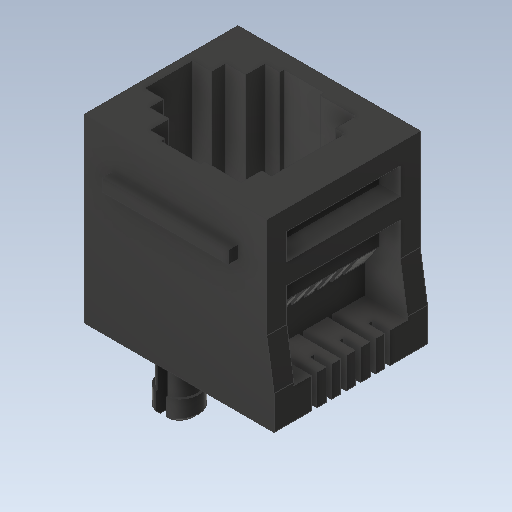
# Autodesk Inventor part: RJ12 - Straight
Saved by Autodesk Inventor 2020 (Build 240168000, 168)
## iProperties
Created: 2017-10-30
Part Number: RJ12 - Straight
Material: Thermoplastic Resin
Document SubType Name: Modeling
Designer: Alex
Density: 1.28 g/cm^3
Appearance: Smooth - Black
Mass: 2.13301 g
Surface Area: 25.086 cm^2
Volume: 1.66642 cm^3
Catalog Web Link: https://www.digikey.com/product-detail/en/assmann-wsw-components/A-2014-1-4-N-T-R/AE10395-ND/2183646
Description: Board Mount RJ12 - Straight
Vendor: Digikey
Author: Alex
Autodesk Inventor part; units mm, degrees
ref_plane "YZ Plane" through (0, 0, 0) normal (1, 0, 0) x (0, 1, 0)
sketch "Sketch1" plane through (0, 0, 0) normal (0, 1, 0) x (-1, 0, 0)
  line L0 (7.9375, -6.6802) -> (-7.9375, -6.6802)
  line L1 (-7.9375, -6.6802) -> (-7.9375, 6.6802)
  line L2 (-7.9375, 6.6802) -> (7.9375, 6.6802)
  line L3 (7.9375, 6.6802) -> (7.9375, -6.6802)
  line L4 (7.9375, -6.6802) -> (-7.9375, 6.6802) construction
  line L5 (-7.9375, -6.6802) -> (7.9375, 6.6802) construction
  point P0 (0, 0)
  dimension "d0" = 15.875
  dimension "d1" = 13.3604
  constraints: 12 end point, 2 midpoint, 2 parallel, 1 horizontal, 1 perpendicular
  measures "d0" distance of L1.end L2.end
  measures "d1" distance of L0.end L1.end
extrude "Extrusion1" add sketch "Sketch1" along normal blind 15.748
sketch "Sketch2" plane through (-7.9375, 0, 6.6802) normal (0, 0, 1) x (1, 0, 0)
  line L0 (15.875, 0) -> (15.875, 15.748) projected
  line L1 (15.875, 0) -> (16.51, 0)
  line L2 (16.51, 0) -> (16.51, 2.921)
  line L3 (16.51, 2.921) -> (15.875, 6.9596)
  line L4 (15.875, 0) -> (15.875, 6.9596)
  line L5 (0, 0) -> (0, 15.748) projected
  line L6 (0, 15.748) -> (15.875, 15.748) projected
  point P0 (7.9375, 0)
  dimension "d4" = 16.51
  dimension "d5" = 2.921
  dimension "d6" = 8.7884
  constraints: 8 end point, 1 horizontal, 1 parallel, 1 perpendicular, 1 point on line
  measures "d4" distance between parallel lines of L5 L2
  measures "d5" distance of L1.end L2.end
  measures "d6" distance from line of L6 L3.end
extrude "Extrusion2" add sketch "Sketch2" against normal up to surface (13.3604 mm away)
sketch "Sketch3" plane through (0, 15.748, 0) normal (0, 1, 0) x (1, 0, 0)
  line L0 (-7.3025, -2.1082) -> (-5.6515, -2.1082)
  line L1 (-5.6515, -2.1082) -> (-5.6515, -3.3401)
  line L2 (-5.6515, -3.3401) -> (-3.9243, -3.3401)
  line L3 (-3.9243, -3.3401) -> (-3.9243, -5.0292)
  line L4 (-3.9243, -5.0292) -> (-2.6289, -5.0292)
  line L5 (-2.6289, -5.0292) -> (-2.6289, -5.3975)
  line L6 (-2.6289, -5.3975) -> (0.8763, -5.3975)
  line L7 (0.8763, -5.3975) -> (0.8763, -5.0292)
  line L8 (0.8763, -5.0292) -> (4.0513, -5.0292)
  line L9 (4.0513, -5.0292) -> (4.0513, -3.2131)
  line L10 (4.0513, -3.2131) -> (4.8895, -3.2131)
  line L11 (4.8895, -3.2131) -> (4.8895, 0)
  line L12 (-7.3025, -2.1082) -> (-7.3025, 0)
  line L13 (-7.9375, 6.6802) -> (-7.9375, -6.6802) projected
  line L14 (-7.3025, 0) -> (4.8895, 0) construction
  line L15 (7.9375, -6.6802) -> (7.9375, 6.6802) construction
  line L16 (-7.3025, 2.1082) -> (-5.6515, 2.1082)
  line L17 (-5.6515, 2.1082) -> (-5.6515, 3.3401)
  line L18 (-5.6515, 3.3401) -> (-3.9243, 3.3401)
  line L19 (-3.9243, 3.3401) -> (-3.9243, 5.0292)
  line L20 (-3.9243, 5.0292) -> (-2.6289, 5.0292)
  line L21 (-2.6289, 5.0292) -> (-2.6289, 5.3975)
  line L22 (-2.6289, 5.3975) -> (0.8763, 5.3975)
  line L23 (0.8763, 5.3975) -> (0.8763, 5.0292)
  line L24 (0.8763, 5.0292) -> (4.0513, 5.0292)
  line L25 (4.0513, 5.0292) -> (4.0513, 3.2131)
  line L26 (4.0513, 3.2131) -> (4.8895, 3.2131)
  line L27 (4.8895, 3.2131) -> (4.8895, 0)
  line L28 (-7.3025, 2.1082) -> (-7.3025, 0)
  point P0 (0, 0)
  dimension "d9" = 0.635
  dimension "d10" = 2.1082
  dimension "d11" = 3.048
  dimension "d12" = 0.8382
  dimension "d13" = 3.175
  dimension "d14" = 3.2131
  dimension "d15" = 5.0292
  dimension "d16" = 5.3975
  dimension "d17" = 1.651
  dimension "d18" = 1.7272
  dimension "d19" = 1.2954
  dimension "d20" = 3.5052
  dimension "d21" = 3.3401
  constraints: 54 end point, 12 symmetric about line, 11 perpendicular, 5 point on line, 1 horizontal, 1 parallel
  measures "d9" distance between parallel lines of L13 L12
  measures "d10" distance between parallel lines of L14 L0
  measures "d11" distance between parallel lines of L15 L11
  measures "d12" distance of L9.end L10.end
  measures "d13" distance of L7.end L8.end
  measures "d14" distance between parallel lines of L14 L10
  measures "d15" distance between parallel lines of L14 L8
  measures "d16" distance between parallel lines of L14 L6
  measures "d17" distance of L0.start L0.end
  measures "d18" distance of L1.end L2.end
  measures "d19" distance of L3.end L4.end
  measures "d20" distance of L5.end L6.end
  measures "d21" distance between parallel lines of L14 L2
extrude "Extrusion3" cut sketch "Sketch3" against normal blind 13.97
sketch "Sketch4" plane through (0, 0, 0) normal (1, 0, 0) x (0, 1, 0)
  line L0 (0, 6.6802) -> (15.748, 6.6802) projected
  line L1 (11.5316, 6.6802) -> (12.6492, 6.6802)
  line L2 (12.6492, 6.6802) -> (12.6492, 7.5692)
  line L3 (12.6492, 7.5692) -> (11.5316, 7.5692)
  line L4 (11.5316, 7.5692) -> (11.5316, 6.6802)
  line L5 (15.748, -6.6802) -> (15.748, 6.6802) projected
  line L6 (0, 0) -> (24.5058, 0) construction
  line L7 (11.5316, -6.6802) -> (12.6492, -6.6802)
  line L8 (12.6492, -6.6802) -> (12.6492, -7.5692)
  line L9 (12.6492, -7.5692) -> (11.5316, -7.5692)
  line L10 (11.5316, -7.5692) -> (11.5316, -6.6802)
  dimension "d24" = 1.1176
  dimension "d25" = 3.0988
  dimension "d27" = 7.5692
  constraints: 18 end point, 4 symmetric about line, 2 horizontal, 2 parallel, 1 perpendicular, 1 point on line
  measures "d24" distance of L2.end L3.end
  measures "d25" distance between parallel lines of L5 L2
  measures "d27" distance between parallel lines of L6 L3
extrude "Extrusion4" add sketch "Sketch4" along normal mid plane 10.922
sketch "Sketch5" plane through (0, 0, 0) normal (0, -1, 0) x (1, 0, 0)
  line L0 (-3.2893, 2.8702) -> (3.5687, 2.8702)
  line L1 (3.5687, 2.8702) -> (3.5687, 2.3622)
  line L2 (3.5687, 2.3622) -> (-3.2893, 2.3622)
  line L3 (-3.2893, 2.3622) -> (-3.2893, 2.8702)
  line L4 (8.5725, 6.6802) -> (-7.9375, 6.6802) projected
  line L5 (-7.9375, 6.6802) -> (-7.9375, -6.6802) projected
  line L6 (-3.2893, 1.8542) -> (3.5687, 1.8542)
  line L7 (3.5687, 1.8542) -> (3.5687, 1.3462)
  line L8 (3.5687, 1.3462) -> (-3.2893, 1.3462)
  line L9 (-3.2893, 1.3462) -> (-3.2893, 1.8542)
  line L10 (-3.2893, 0.8382) -> (3.5687, 0.8382)
  line L11 (3.5687, 0.8382) -> (3.5687, 0.3302)
  line L12 (3.5687, 0.3302) -> (-3.2893, 0.3302)
  line L13 (-3.2893, 0.3302) -> (-3.2893, 0.8382)
  line L14 (-3.2893, -0.1778) -> (3.5687, -0.1778)
  line L15 (3.5687, -0.1778) -> (3.5687, -0.6858)
  line L16 (3.5687, -0.6858) -> (-3.2893, -0.6858)
  line L17 (-3.2893, -0.6858) -> (-3.2893, -0.1778)
  line L18 (-3.2893, -1.1938) -> (3.5687, -1.1938)
  line L19 (3.5687, -1.1938) -> (3.5687, -1.7018)
  line L20 (3.5687, -1.7018) -> (-3.2893, -1.7018)
  line L21 (-3.2893, -1.7018) -> (-3.2893, -1.1938)
  line L22 (-3.2893, -2.2098) -> (3.5687, -2.2098)
  line L23 (3.5687, -2.2098) -> (3.5687, -2.7178)
  line L24 (3.5687, -2.7178) -> (-3.2893, -2.7178)
  line L25 (-3.2893, -2.7178) -> (-3.2893, -2.2098)
  line L26 (8.5725, 6.6802) -> (8.5725, -6.6802) projected
  line L27 (-7.3025, 2.1082) -> (-7.3025, -2.1082) projected
  line L28 (-7.3025, -2.1082) -> (-5.6515, -2.1082) projected
  line L29 (-5.6515, 2.1082) -> (-7.3025, 2.1082) projected
  line L30 (-5.6515, -2.1082) -> (-5.6515, 2.1082)
  point P0 (0, 0)
  point P1 (7.9375, 6.6802)
  dimension "d30" = 0.508
  dimension "d31" = 6.858
  dimension "d32" = 3.81
  dimension "d36" = 1.016
  dimension "d41" = 5.0038
  constraints: 50 end point, 2 parallel, 2 perpendicular, 1 horizontal, 1 vertical, 40 other
  measures "d30" distance of L2.end L0.start
  measures "d31" distance of L0.start L0.end
  measures "d32" distance between parallel lines of L4 L0
  measures "d36" distance of L0.start L6.start
  measures "d41" distance between parallel lines of L26 L1
extrude "Extrusion5" cut sketch "Sketch5" against normal up to next
sketch "Sketch6" plane through (0, 0, 0) normal (0, -1, 0) x (1, 0, 0)
  circle A0 centre (-4.2291, 4.826) radius 0.9207
  circle A1 centre (-4.2291, -4.826) radius 0.9207
  line L0 (-7.9375, 6.6802) -> (-7.9375, -6.6802) projected
  line L1 (8.5725, 6.6802) -> (-7.9375, 6.6802) projected
  line L2 (-7.9375, -6.6802) -> (8.5725, -6.6802) projected
  point P0 (0, 0)
  point P1 (7.9375, 6.6802)
  point P2 (7.9375, -6.6802)
  dimension "d44" = 3.7084
  dimension "d45" = 1.8542
  dimension "d46" = 1.8415
  dimension "d47" = 1.8542
  constraints: 2 centre point, 1 equal radius, 1 vertical alignment
  measures "d44" distance from line of L0 A0.centre
  measures "d45" distance from line of L1 A0.centre
  measures "d46" diameter of A0
  measures "d47" distance from line of L2 A1.centre
extrude "Extrusion6" cut sketch "Sketch6" against normal blind 1.27
ref_plane "Work Plane1" through (0, 0, 4.9213) normal (0, 0, 1) x (1, 0, 0)
ref_plane "Work Plane2" through (0, 0, -4.9213) normal (0, 0, 1) x (1, 0, 0)
sketch "Sketch7" plane through (0, 0, 4.9213) normal (0, 0, 1) x (1, 0, 0)
  line L0 (3.5687, 0) -> (-3.2893, 0) projected
  line L1 (-2.9591, 0) -> (-2.9591, -2.1844)
  line L2 (-2.9591, -2.1844) -> (-3.1115, -2.1844)
  line L3 (-3.1115, -2.1844) -> (-3.1115, -3.6576)
  line L4 (-3.1115, -3.6576) -> (-2.7051, -4.064)
  line L5 (-2.7051, -4.064) -> (-1.4351, -4.064)
  line L6 (-1.4351, -4.064) -> (-1.4351, 0)
  line L7 (-2.9591, 0) -> (-1.4351, 0)
  line L8 (-7.9375, 0) -> (-7.9375, 15.748) projected
  point P0 (0, 0)
  dimension "d52" = 1.524
  dimension "d53" = 4.9784
  dimension "d54" = 1.6764
  dimension "d55" = 45
  dimension "d56" = 1.27
  dimension "d57" = 4.064
  dimension "d58" = 2.1844
  constraints: 14 end point, 4 point on line, 3 perpendicular, 1 parallel, 1 vertical
  measures "d52" distance between parallel lines of L6 L1
  measures "d53" distance between parallel lines of L8 L1
  measures "d54" distance between parallel lines of L6 L3
  measures "d55" angle of L3 L4
  measures "d56" distance from line of L6 L4.end
  measures "d57" distance between parallel lines of L0 L5
  measures "d58" distance of L1.start L1.end
revolve "Revolution1" add sketch "Sketch7" angle 360 about axis through (-1.4351, -4.064, 4.9213) along (0, 1, 0)
sketch "Sketch8" plane through (0, 0, -4.9213) normal (0, 0, 1) x (1, 0, 0)
  line L0 (-2.9591, 0) -> (-2.9591, -2.1844)
  line L1 (-2.9591, -2.1844) -> (-3.1115, -2.1844)
  line L2 (-3.1115, -2.1844) -> (-3.1115, -3.6576)
  line L3 (-3.1115, -3.6576) -> (-2.7051, -4.064)
  line L4 (-2.7051, -4.064) -> (-1.4351, -4.064)
  line L5 (-1.4351, -4.064) -> (-1.4351, 0)
  line L6 (-2.9591, 0) -> (-1.4351, 0)
  line L7 (-7.9375, 0) -> (-7.9375, 15.748)
  point P0 (0, 0)
  point P1 (0, 0)
  dimension "d60" = 1.524
  dimension "d61" = 4.9784
  dimension "d62" = 1.6764
  dimension "d63" = 45
  dimension "d64" = 1.27
  dimension "d66" = 2.1844
  constraints: 16 end point, 3 perpendicular, 1 parallel, 1 point on line, 1 vertical
  measures "d60" distance between parallel lines of L5 L0
  measures "d61" distance between parallel lines of L7 L0
  measures "d62" distance between parallel lines of L5 L2
  measures "d63" angle of L2 L3
  measures "d64" distance from line of L5 L3.end
  measures "d66" distance of L0.start L0.end
revolve "Revolution2" add sketch "Sketch8" angle 360 about axis through (-1.4351, -4.064, -4.9213) along (0, 1, 0)
sketch "Sketch9" plane through (-1.4351, -4.064, 4.9213) normal (0, -1, 0) x (1, 0, 0)
  line L0 (-0.4572, 1.6764) -> (0.4572, 1.6764)
  line L1 (0.4572, 1.6764) -> (0.4572, -11.5189)
  line L2 (0.4572, -11.5189) -> (-0.4572, -11.5189)
  line L3 (-0.4572, -11.5189) -> (-0.4572, 1.6764)
  circle A0 centre (0, 0) radius 1.6764 construction
  circle A1 centre (0, -9.8425) radius 1.6764 construction
  point P0 (1.4351, -4.9213)
  point P1 (0, 1.6764)
  point P2 (0, -11.5189)
  dimension "d68" = 0.9144
  constraints: 8 end point, 3 vertical alignment, 2 midpoint, 2 parallel, 1 horizontal, 1 perpendicular, 2 other
  measures "d68" distance between parallel lines of L1 L3
extrude "Extrusion7" cut sketch "Sketch9" against normal up to surface (4.064 mm away)
sketch "Sketch10" plane through (0, 0, 0) normal (0, 0, 1) x (1, 0, 0)
  line L0 (7.9375, 6.9596) -> (7.9375, 15.748) projected
  line L1 (7.9375, 13.97) -> (6.1595, 13.97)
  line L2 (6.1595, 13.97) -> (6.1595, 11.684)
  line L3 (6.1595, 11.684) -> (7.9375, 11.684)
  line L4 (7.9375, 11.684) -> (7.9375, 13.97)
  line L5 (7.9375, 15.748) -> (-7.9375, 15.748) projected
  line L6 (8.5725, 0) -> (8.5725, 2.921) projected
  line L7 (8.5725, 2.667) -> (4.5593, 2.667)
  line L8 (4.5593, 2.667) -> (4.5593, 4.699)
  line L9 (4.5593, 4.699) -> (6.096, 6.9596)
  line L10 (6.096, 6.9596) -> (6.096, 9.8806)
  line L11 (6.096, 9.8806) -> (8.5725, 9.8806)
  line L12 (8.5725, 9.8806) -> (8.5725, 2.667)
  line L13 (-7.9375, 0) -> (8.5725, 0) projected
  point P0 (0, 0)
  point P1 (7.9375, 0)
  dimension "d71" = 1.778
  dimension "d72" = 2.286
  dimension "d73" = 1.778
  dimension "d74" = 2.921
  dimension "d75" = 1.8034
  dimension "d76" = 2.667
  dimension "d77" = 4.0132
  dimension "d78" = 2.032
  dimension "d79" = 1.8415
  constraints: 20 end point, 5 perpendicular, 3 parallel, 2 point on line, 1 horizontal
  measures "d71" distance between parallel lines of L5 L1
  measures "d72" distance of L1.end L2.end
  measures "d73" distance of L2.end L3.end
  measures "d74" distance of L9.end L10.end
  measures "d75" distance between parallel lines of L3 L11
  measures "d76" distance between parallel lines of L13 L7
  measures "d77" distance of L7.start L7.end
  measures "d78" distance of L7.end L8.end
  measures "d79" distance between parallel lines of L10 L0
extrude "Extrusion8" cut sketch "Sketch10" along normal mid plane 9.8806
sketch "Sketch11" plane through (0, 0, 0) normal (0, -1, 0) x (1, 0, 0)
  line L0 (8.5725, 6.6802) -> (8.5725, -6.6802) projected
  line L1 (8.5725, 3.4036) -> (4.4831, 3.4036)
  line L2 (4.4831, 3.4036) -> (4.4831, 2.9464)
  line L3 (4.4831, 2.9464) -> (8.5725, 2.9464)
  line L4 (8.5725, 2.9464) -> (8.5725, 3.4036)
  line L5 (8.5725, 6.6802) -> (-7.9375, 6.6802) projected
  line L6 (8.5725, 0.8636) -> (4.4831, 0.8636)
  line L7 (4.4831, 0.8636) -> (4.4831, 0.4064)
  line L8 (4.4831, 0.4064) -> (8.5725, 0.4064)
  line L9 (8.5725, 0.4064) -> (8.5725, 0.8636)
  line L10 (8.5725, -1.6764) -> (4.4831, -1.6764)
  line L11 (4.4831, -1.6764) -> (4.4831, -2.1336)
  line L12 (4.4831, -2.1336) -> (8.5725, -2.1336)
  line L13 (8.5725, -2.1336) -> (8.5725, -1.6764)
  line L14 (8.5725, 2.1336) -> (7.0993, 2.1336)
  line L15 (7.0993, 2.1336) -> (7.0993, 1.6764)
  line L16 (7.0993, 1.6764) -> (8.5725, 1.6764)
  line L17 (8.5725, 1.6764) -> (8.5725, 2.1336)
  line L18 (7.0993, -0.8636) -> (8.5725, -0.8636)
  line L19 (7.0993, -0.4064) -> (7.0993, -0.8636)
  line L20 (8.5725, -0.8636) -> (8.5725, -0.4064)
  line L21 (8.5725, -0.4064) -> (7.0993, -0.4064)
  line L22 (7.0993, -3.4036) -> (8.5725, -3.4036)
  line L23 (7.0993, -2.9464) -> (7.0993, -3.4036)
  line L24 (8.5725, -3.4036) -> (8.5725, -2.9464)
  line L25 (8.5725, -2.9464) -> (7.0993, -2.9464)
  point P0 (0, 0)
  point P1 (7.9375, 6.6802)
  dimension "d82" = 0.4572
  dimension "d83" = 3.2766
  dimension "d84" = 4.0894
  dimension "d87" = 2.54
  dimension "d92" = 1.27
  dimension "d93" = 1.4732
  dimension "d96" = 2.54
  constraints: 48 end point, 5 parallel, 2 horizontal, 2 perpendicular, 2 point on line, 2 vertical, 32 other
  measures "d82" distance of L1.end L2.end
  measures "d83" distance between parallel lines of L5 L1
  measures "d84" distance of L2.end L3.end
  measures "d87" distance of L1.start L6.start
  measures "d92" distance between parallel lines of L1 L14
  measures "d93" distance of L14.start L14.end
  measures "d96" distance of L15.end L18.start
extrude "Extrusion9" cut sketch "Sketch11" against normal up to surface (2.667 mm away)
sketch "Sketch12" plane through (6.096, 6.9596, -4.9403) normal (1, 0, 0) x (0, 0, -1)
  line L0 (-8.1534, -1.7749) -> (-8.1534, -2.2606) construction
  line L1 (-1.7272, -1.7749) -> (-8.1534, -1.7749) construction
  line L2 (-1.7272, -2.2606) -> (-1.7272, -1.7749) construction
  line L3 (-1.7272, -2.2606) -> (0, -2.2606) construction
  line L4 (0, -2.2606) -> (0, 0) construction
  line L5 (-9.8806, 0) -> (0, 0) construction
  line L6 (-9.8806, 0) -> (-9.8806, -2.2606) construction
  line L7 (-9.8806, -2.2606) -> (-8.1534, -2.2606) construction
  line L8 (-8.1026, 0) -> (-7.5946, 0)
  line L9 (-7.5946, 0) -> (-7.5946, -1.7749)
  line L10 (-7.5946, -1.7749) -> (-8.1026, -1.7749)
  line L11 (-8.1026, -1.7749) -> (-8.1026, 0)
  line L12 (-6.9545, 0) -> (-6.4465, 0)
  line L13 (-6.4465, 0) -> (-6.4465, -1.7749)
  line L14 (-6.4465, -1.7749) -> (-6.9545, -1.7749)
  line L15 (-6.9545, -1.7749) -> (-6.9545, 0)
  line L16 (-5.8064, 0) -> (-5.2984, 0)
  line L17 (-5.2984, 0) -> (-5.2984, -1.7749)
  line L18 (-5.2984, -1.7749) -> (-5.8064, -1.7749)
  line L19 (-5.8064, -1.7749) -> (-5.8064, 0)
  line L20 (-4.6584, 0) -> (-4.1504, 0)
  line L21 (-4.1504, 0) -> (-4.1504, -1.7749)
  line L22 (-4.1504, -1.7749) -> (-4.6584, -1.7749)
  line L23 (-4.6584, -1.7749) -> (-4.6584, 0)
  line L24 (-3.5103, 0) -> (-3.0023, 0)
  line L25 (-3.0023, 0) -> (-3.0023, -1.7749)
  line L26 (-3.0023, -1.7749) -> (-3.5103, -1.7749)
  line L27 (-3.5103, -1.7749) -> (-3.5103, 0)
  line L28 (-2.3622, 0) -> (-1.8542, 0)
  line L29 (-1.8542, 0) -> (-1.8542, -1.7749)
  line L30 (-1.8542, -1.7749) -> (-2.3622, -1.7749)
  line L31 (-2.3622, -1.7749) -> (-2.3622, 0)
  point P0 (-4.9403, -6.9596)
  point P1 (-7.0053, -1.7749)
  point P2 (-5.8572, -1.7749)
  point P3 (-4.7092, -1.7749)
  point P4 (-3.5611, -1.7749)
  point P5 (-2.413, -1.7749)
  dimension "d103" = 0.508
  dimension "d105" = 1.778
  dimension "d108" = 1.1481
  constraints: 48 end point, 2 horizontal, 2 parallel, 2 point on line, 1 perpendicular, 45 other
  measures "d103" distance of L9.end L10.end
  measures "d105" distance between parallel lines of L6 L11
  measures "d108" distance of L0.start point (-7.005, -1.775)
extrude "Extrusion10" cut sketch "Sketch12" against normal up to surface (1.2065 mm away)
sketch "Sketch13" plane through (0, 0, 0) normal (0, 0, 1) x (1, 0, 0)
  line L0 (4.8895, 5.1847) -> (4.8895, 6.9596) projected
  line L1 (4.8895, 2.667) -> (8.5725, 2.667) projected
  line L2 (4.0513, 1.778) -> (4.8895, 1.778) projected
  line L3 (4.0513, 15.748) -> (4.8895, 15.748) projected
  line L4 (0.8763, 1.778) -> (4.0513, 1.778) projected
  line L5 (4.0513, 1.778) -> (4.0513, 4.5867)
  line L6 (4.0513, 15.748) -> (4.0513, 1.778) projected
  line L7 (4.0513, 4.5867) -> (4.8895, 5.8197)
  line L8 (4.8895, 5.8197) -> (4.8895, 1.778)
  line L9 (4.8895, 5.1847) -> (6.096, 6.9596) projected
  point P0 (0, 0)
  point P1 (7.9375, 2.667)
  dimension "d115" = 0.635
  constraints: 6 end point, 2 point on line, 1 collinear, 1 parallel
  measures "d115" distance of L0.start L7.end
extrude "Extrusion11" add sketch "Sketch13" along normal mid plane 10.16
equation "\"d36\" = 2 * d30"
equation "\"d47\" = d45"
body "Solid1"
